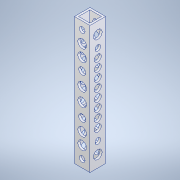
# Autodesk Inventor part: ハンド9x9_3
Saved by Autodesk Inventor 2020.3 (Build 243373000, 373)
## iProperties
Created: 2020-05-31
Part Number: ハンド9x9_3
Material: アルミニウム 6061
Document SubType Name: Modeling
Designer: totot
Density: 2.7 g/cm^3
Appearance: アルミニウム - フラット
Mass: 5.3761 g
Surface Area: 40.9617 cm^2
Volume: 1.99115 cm^3
Author: totot
Autodesk Inventor part; units mm, degrees
ref_plane "YZ Plane" through (0, 0, 0) normal (1, 0, 0) x (0, 1, 0)
ref_plane "XZ Plane" through (0, 0, 0) normal (0, 1, 0) x (-1, 0, 0)
ref_plane "XY Plane" through (0, 0, 0) normal (0, 0, 1) x (1, 0, 0)
sketch "スケッチ1" plane through (0, 0, 0) normal (0, 1, 0) x (-1, 0, 0)
  line L0 (0, 0) -> (-9, 0)
  line L1 (-9, 0) -> (-9, 9)
  line L2 (-9, 9) -> (0, 9)
  line L3 (0, 9) -> (0, 0)
  line L4 (-1.2, 7.8) -> (-7.8, 7.8)
  line L5 (-7.8, 7.8) -> (-7.8, 1.2)
  line L6 (-7.8, 1.2) -> (-1.2, 1.2)
  line L7 (-1.2, 1.2) -> (-1.2, 7.8)
  dimension "d0" = 9
  dimension "d1" = 9
  dimension "d2" = 1.2
  dimension "d3" = 1.2
  dimension "d4" = 1.2
  dimension "d5" = 1.2
  constraints: 16 end point, 4 parallel, 2 horizontal, 2 perpendicular
  measures "d0" distance of L1.end L2.end
  measures "d1" distance of L0.end L1.end
  measures "d2" distance between parallel lines of L2 L4
  measures "d3" distance between parallel lines of L0 L6
  measures "d4" distance between parallel lines of L7 L3
  measures "d5" distance between parallel lines of L1 L5
extrude "押し出し1" add sketch "スケッチ1" along normal blind 73.5
sketch "スケッチ2" plane through (0, 0, 9) normal (0, 0, 1) x (1, 0, 0)
  line L0 (0, 0) -> (0, 73.5) projected
  line L1 (0, 0) -> (9, 0) projected
  line L2 (0, 73.5) -> (9, 73.5) projected
  point P0 (4.5, 69)
  point P1 (4.5, 4.5)
  dimension "d8" = 4.5
  dimension "d9" = 4.5
  dimension "d10" = 4.5
  dimension "d11" = 4.5
  measures "d8" distance from line of L0 point (4.5, 69)
  measures "d9" distance from line of L0 point (4.5, 4.5)
  measures "d10" distance from line of L1 point (4.5, 4.5)
  measures "d11" distance from line of point (4.5, 69) L2
hole "穴1" at (4.5, 69, 9) at (4.5, 4.5, 9) direction (0, 0, -1) diameter 3.3 end through all
sketch "スケッチ3" plane through (9, 0, 9) normal (1, 0, 0) x (0, 0, -1)
  line L0 (0, 0) -> (0, 73.5) projected
  line L1 (0, 73.5) -> (9, 73.5) projected
  line L2 (0, 0) -> (9, 0) projected
  point P0 (4.5, 60)
  point P1 (4.5, 13.5)
  dimension "d19" = 4.5
  dimension "d20" = 4.5
  dimension "d21" = 13.5
  dimension "d22" = 13.5
  measures "d19" distance from line of L0 point (4.5, 60)
  measures "d20" distance from line of L0 point (4.5, 13.5)
  measures "d21" distance from line of point (4.5, 60) L1
  measures "d22" distance from line of point (4.5, 13.5) L2
hole "穴2" at (9, 60, 4.5) at (9, 13.5, 4.5) direction (-1, 0, 0) diameter 3.3 end through all
sketch "スケッチ4" plane through (9, 0, 0) normal (0, 0, -1) x (-1, 0, 0)
  line L0 (9, 0) -> (9, 73.5) projected
  line L1 (0, 73.5) -> (9, 73.5) projected
  line L2 (0, 0) -> (9, 0) projected
  point P0 (4.5, 48.5)
  point P1 (4.5, 25)
  dimension "d30" = 4.5
  dimension "d31" = 4.5
  dimension "d32" = 25
  dimension "d33" = 25
  measures "d30" distance from line of point (4.5, 48.5) L0
  measures "d31" distance from line of L0 point (4.5, 25)
  measures "d32" distance from line of point (4.5, 48.5) L1
  measures "d33" distance from line of point (4.5, 25) L2
hole "穴3" at (4.5, 48.5, 0) at (4.5, 25, 0) direction (0, 0, 1) diameter 4 end through all
sketch "スケッチ5" plane through (0, 0, 9) normal (0, 0, 1) x (1, 0, 0)
  circle A0 centre (4.5, 25) radius 2 projected
  circle A1 centre (4.5, 4.5) radius 1.65 projected
  circle A2 centre (4.5, 48.5) radius 2 projected
  line L0 (0, 0) -> (0, 73.5) projected
  point P0 (4.5, 11.3333)
  point P1 (4.5, 18.1667)
  point P2 (4.5, 32.8333)
  point P3 (4.5, 55.3333)
  point P4 (4.5, 62.1667)
  point P5 (4.5, 40.6667)
  dimension "d41" = 20.5
  dimension "d42" = 23.5
  dimension "d43" = 4.5
  dimension "d44" = 4.5
  dimension "d45" = 6.8333
  dimension "d46" = 6.8333
  dimension "d47" = 4.5
  dimension "d48" = 7.8333
  dimension "d49" = 7.8333
  dimension "d50" = 6.8333
  dimension "d51" = 6.8333
  dimension "d52" = 4.5
  dimension "d53" = 4.5
  dimension "d54" = 4.5
  measures "d41" distance of A0.centre A1.centre
  measures "d42" distance of A2.centre A0.centre
  measures "d43" distance from line of point (4.5, 11.333) L0
  measures "d44" distance from line of L0 point (4.5, 18.167)
  measures "d45" distance of point (4.5, 11.333) A1.centre
  measures "d46" distance of point (4.5, 18.167) point (4.5, 11.333)
  measures "d47" distance from line of L0 point (4.5, 32.833)
  measures "d48" distance of point (4.5, 32.833) A0.centre
  measures "d49" distance of point (4.5, 40.667) point (4.5, 32.833)
  measures "d50" distance of A2.centre point (4.5, 55.333)
  measures "d51" distance of point (4.5, 55.333) point (4.5, 62.167)
  measures "d52" distance from line of point (4.5, 55.333) L0
  measures "d53" distance from line of L0 point (4.5, 62.167)
  measures "d54" distance from line of L0 point (4.5, 40.667)
hole "穴4" at (4.5, 11.3333, 9) at (4.5, 18.1667, 9) at (4.5, 32.8333, 9) at (4.5, 55.3333, 9) at (4.5, 62.1667, 9) at (4.5, 40.6667, 9) direction (0, 0, -1) diameter 5 end through all
sketch "スケッチ6" plane through (0, 0, 0) normal (-1, 0, 0) x (0, 0, 1)
  line L0 (9, 0) -> (9, 73.5) projected
  circle A0 centre (4.5, 13.5) radius 1.65 projected
  line L1 (0, 0) -> (9, 0) projected
  circle A1 centre (4.5, 60) radius 1.65 projected
  point P0 (4.5, 66.75)
  point P1 (4.5, 6.75)
  dimension "d62" = 4.5
  dimension "d63" = 4.5
  dimension "d64" = 13.5
  dimension "d65" = 6.75
  dimension "d66" = 6.75
  measures "d62" distance from line of point (4.5, 66.75) L0
  measures "d63" distance from line of point (4.5, 6.75) L0
  measures "d64" distance from line of A0.centre L1
  measures "d65" distance from line of point (4.5, 6.75) L1
  measures "d66" distance of A1.centre point (4.5, 66.75)
hole "穴5" at (0, 66.75, 4.5) at (0, 6.75, 4.5) direction (1, 0, 0) diameter 5 end through all
sketch "スケッチ7" plane through (0, 0, 0) normal (-1, 0, 0) x (0, 0, 1)
  line L0 (9, 0) -> (9, 73.5) projected
  circle A0 centre (4.5, 60) radius 1.65 projected
  point P0 (0, 0)
  point P1 (4.5, 54.9649)
  point P2 (4.5, 49.9649)
  point P3 (4.5, 44.9649)
  point P4 (4.5, 39.9649)
  point P5 (4.5, 34.9649)
  point P6 (4.5, 29.9649)
  point P7 (4.5, 24.9649)
  point P8 (4.5, 19.9649)
  dimension "d74" = 4.5
  dimension "d75" = 5.0351
  dimension "d78" = 5
  constraints: 1 vertical, 7 other
  measures "d74" distance from line of point (4.5, 54.965) L0
  measures "d75" distance of point (4.5, 54.965) A0.centre
  measures "d78" distance of point (4.5, 54.965) point (4.5, 49.965)
hole "穴6" at (0, 54.9649, 4.5) at (0, 49.9649, 4.5) at (0, 44.9649, 4.5) at (0, 39.9649, 4.5) at (0, 34.9649, 4.5) at (0, 29.9649, 4.5) at (0, 24.9649, 4.5) at (0, 19.9649, 4.5) direction (1, 0, 0) diameter 4 end through all
equation "\"d3\" = d2"
equation "\"d4\" = d3"
equation "\"d5\" = d4"
equation "\"d9\" = d8"
equation "\"d10\" = d9"
equation "\"d11\" = d8"
equation "\"d20\" = d19"
equation "\"d22\" = d21"
equation "\"d33\" = d32"
equation "\"d44\" = d43"
equation "\"d45\" = 0.333333 * d41"
equation "\"d46\" = d45"
equation "\"d47\" = d44"
equation "\"d48\" = 0.333333 * d42"
equation "\"d49\" = d48"
equation "\"d50\" = d46"
equation "\"d51\" = d50"
equation "\"d52\" = d47"
equation "\"d53\" = d52"
equation "\"d54\" = d47"
equation "\"d63\" = d62"
equation "\"d65\" = 0.5 * d64"
equation "\"d66\" = d65"
